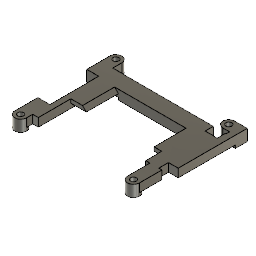
picooler (Autodesk Fusion 360 design; units mm, degrees)
Autodesk Fusion 360 part; units mm, degrees
sketch "Skizze1" plane through (0, 0, 0) normal (0, 0, 1) x (1, 0, 0)
  line L0 (0, 0) -> (65, 0)
  line L1 (65, 0) -> (65, 56)
  line L2 (65, 56) -> (0, 56)
  line L3 (0, 56) -> (0, 0)
  circle A0 centre (61.5, 52.5) radius 1.5
  circle A1 centre (3.5, 52.5) radius 1.5
  circle A2 centre (3.5, 3.5) radius 1.5
  circle A3 centre (61.5, 3.5) radius 1.5
  line L4 (3.5, 3.5) -> (61.5, 3.5) construction
  line L5 (61.5, 3.5) -> (61.5, 52.5) construction
  line L6 (61.5, 52.5) -> (3.5, 52.5) construction
  line L7 (3.5, 52.5) -> (3.5, 3.5) construction
  line L8 (9.5, 39.8) -> (56.2, 39.8) construction
  line L9 (56.2, 39.8) -> (56.2, 23.3) construction
  line L10 (56.2, 23.3) -> (9.5, 23.3) construction
  line L11 (9.5, 23.3) -> (9.5, 39.8) construction
  line L12 (18.5, 39.8) -> (18.5, 35.3) construction
  line L13 (18.5, 35.3) -> (9.5, 35.3) construction
  line L14 (19.5, 25) -> (33.5, 25) construction
  line L15 (33.5, 25) -> (33.5, 39) construction
  line L16 (33.5, 39) -> (19.5, 39) construction
  line L17 (19.5, 39) -> (19.5, 25) construction
  line L18 (7, 49.3) -> (17.5, 49.3) construction
  line L19 (17.5, 49.3) -> (17.5, 36.3) construction
  line L20 (17.5, 36.3) -> (7, 36.3) construction
  line L21 (7, 36.3) -> (7, 49.3) construction
  line L22 (52.2, 39.8) -> (52.2, 23.3) construction
  line L23 (17.5, 23.3) -> (17.5, 36.3) construction
  circle A4 centre (3.5, 52.5) radius 3.1
  circle A5 centre (61.5, 52.5) radius 3.1
  circle A6 centre (3.5, 3.5) radius 3.1
  circle A7 centre (61.5, 3.5) radius 3.1
  line L24 (6.6, 52.5) -> (0.4, 52.5) construction
  line L25 (0.4, 52.5) -> (0.4, 40.5)
  line L26 (0.4, 40.5) -> (6.6, 40.5)
  line L27 (6.6, 40.5) -> (6.6, 52.5)
  line L28 (61.5, 49.4) -> (68, 49.4)
  line L29 (68, 49.4) -> (68, 55.6)
  line L30 (68, 55.6) -> (61.5, 55.6)
  line L31 (61.5, 55.6) -> (61.5, 49.4) construction
  dimension "d1" = 65
  dimension "d2" = 56
  dimension "d3" = 49
  dimension "d4" = 3.5
  dimension "d5" = 4
  dimension "d6" = 3.5
  dimension "d7" = 3.5
  dimension "d8" = 3
  dimension "d9" = 3
  dimension "d10" = 3
  dimension "d11" = 3
  dimension "d12" = 46.7
  dimension "d13" = 16.5
  dimension "d14" = 4.5
  dimension "d15" = 9
  dimension "d16" = 14
  dimension "d17" = 14
  dimension "d18" = 17
  dimension "d19" = 19.5
  dimension "d20" = 10.5
  dimension "d21" = 13
  dimension "d22" = 6.7
  dimension "d23" = 7
  dimension "d24" = 2
  dimension "d25" = 1
  dimension "d26" = 1
  dimension "d27" = 1
  dimension "d28" = 4
  dimension "d29" = 8
  dimension "d30" = 6.2
  dimension "d31" = 6.2
  dimension "d32" = 6.2
  dimension "d33" = 6.2
  dimension "d36" = 12
  dimension "d37" = 6.5
  measures "d3" distance of L0.start
  measures "d4" distance of L0 L4
  measures "d5" distance of L2 L6
  measures "d6" distance of L1 L5
  measures "d7" distance of L3 L7
  measures "d8" diameter of A1
  measures "d9" diameter of A0
  measures "d10" diameter of A3
  measures "d11" diameter of A2
  measures "d12" distance of L0.start
  measures "d14" distance of L8 L13
  measures "d15" distance of L11 L12
  measures "d16" distance of L0.start
  measures "d17" distance of L14 L16
  measures "d18" distance of L2 L16
  measures "d19" distance of L3 L17
  measures "d22" distance of L2 L18
  measures "d23" distance of L3 L21
  measures "d24" distance of L17 L19
  measures "d25" distance of L12 L19
  measures "d26" distance of L12 L17
  measures "d27" distance of L13 L20
  measures "d28" distance of L9 L22
  measures "d29" distance of L11 L23
  measures "d30" diameter of A4
  measures "d31" diameter of A5
  measures "d32" diameter of A6
  measures "d33" diameter of A7
ref_plane "Arbeitsebene1" through (0, 0, 4) normal (0, 0, 1) x (1, 0, 0)
sketch "Skizze2" plane through (0, 0, 4) normal (0, 0, 1) x (1, 0, 0)
  line L0 (52.2, 39.8) -> (52.2, 23.3)
  line L1 (56.2, 39.8) -> (56.2, 23.3)
  line L2 (56.2, 23.3) -> (9.5, 23.3)
  line L3 (9.5, 39.8) -> (56.2, 39.8)
  line L4 (9.5, 23.3) -> (9.5, 39.8)
  line L5 (17.5, 23.3) -> (17.5, 36.3)
  line L6 (17.5, 49.3) -> (17.5, 36.3)
  line L7 (56.2, 39.8) -> (9.5, 39.8)
  line L8 (9.5, 39.8) -> (9.5, 47.8)
  line L9 (9.5, 47.8) -> (56.2, 47.8)
  line L10 (56.2, 47.8) -> (56.2, 39.8)
  line L11 (56.2, 47.8) -> (68, 47.8)
  line L12 (68, 47.8) -> (68, 15)
  line L13 (68, 15) -> (56.2, 15)
  line L14 (56.2, 15) -> (56.2, 47.8)
  line L15 (0, 0) -> (65, 0)
  line L16 (68, 49.4) -> (68, 55.6)
  line L17 (68, 15) -> (63, 15)
  line L18 (63, 15) -> (63, 20)
  line L19 (63, 20) -> (68, 20)
  line L20 (68, 20) -> (68, 15)
  line L21 (68, 49.4) -> (68, 47.8)
  line L22 (61.5, 49.4) -> (68, 49.4)
  line L23 (65, 0) -> (65, 56)
  line L24 (65, 47.8) -> (65, 49.4)
  line L25 (58.4, 47.8) -> (64.6, 47.8)
  line L26 (64.6, 47.8) -> (64.6, 43.5)
  line L27 (64.6, 43.5) -> (58.4, 43.5)
  line L28 (58.4, 43.5) -> (58.4, 47.8)
  circle A0 centre (61.5, 52.5) radius 3.1
  line L29 (58.4, 15) -> (64.6, 15)
  line L30 (64.6, 15) -> (64.6, 3.5)
  line L31 (64.6, 3.5) -> (58.4, 3.5)
  line L32 (58.4, 3.5) -> (58.4, 15)
  circle A1 centre (61.5, 3.5) radius 3.1
  line L33 (6.6, 40.5) -> (9.5, 40.5)
  line L34 (6.6, 40.5) -> (6.6, 52.5)
  line L35 (9.5, 47.8) -> (6.6, 47.8)
  line L36 (6.6, 3.5) -> (0.4, 3.5)
  line L37 (0.4, 3.5) -> (0.4, 15.5)
  line L38 (0.4, 15.5) -> (6.6, 15.5)
  line L39 (6.6, 15.5) -> (6.6, 3.5)
  circle A2 centre (3.5, 3.5) radius 3.1
  line L40 (3.5, 3.5) -> (61.5, 3.5)
  line L41 (6.6, 40.5) -> (6.6, 15.5)
  line L42 (9.5, 23.3) -> (9.5, 6.6)
  line L43 (6.6, 6.6) -> (9.5, 6.6)
  line L44 (6.6, 36.3) -> (9.5, 36.3)
  dimension "d45" = 8
  dimension "d50" = 15
  dimension "d52" = 20
  dimension "d53" = 5
  dimension "d70" = 9
  dimension "d81" = 12
  measures "d50" distance of L13 L15
  measures "d52" distance of L15 L19
  measures "d53" distance of L12 L18
extrude "Extrusion3" add sketch "Skizze2" along normal blind 2 contours L0 L1 L2 L3 L7 L14 | L2 L3 L4 L5 L6 L7 makes body 1 at (54.8667, 28.8, 4) makes body 2 at (12.1667, 28.8, 4)
chamfer "Fase1" distance 2 angle 45 1 edges at (17.5, 31.55, 6) measured on face at (12.1667, 28.8, 6) on bodies 2
extrude "Extrusion4" add sketch "Skizze2" along normal blind 2 contours L3 L6 L7 L9 L10 L14 | L3 L6 L7 L8 L9 bodies 1 2
extrude "Extrusion5" add sketch "Skizze2" against normal blind 3 contours L3 L6 L7 L9 L10 L14 bodies 1
extrude "Extrusion6" add sketch "Skizze2" along normal blind 2 and the other way blind 2.4 contours L1 L10 L11 L13 L14 L18 L19 L23 L26 L27 L28 L29 | L11 L12 L19 L23 bodies 1
extrude "Extrusion7" add sketch "Skizze1" along normal blind 6 separate body contours L1 A5 L28 L30 | L1 L28 L29 L30 | A5 makes body 3
extrude "Extrusion8" add sketch "Skizze1" along normal blind 6 separate body contours A4 | A4 L25 L26 L27 makes body 4
extrude "Extrusion9" add sketch "Skizze1" along normal blind 6 separate body contours A7 makes body 5
extrude "Extrusion10" add sketch "Skizze1" along normal blind 6 separate body contours A6 makes body 6
extrude "Extrusion11" add sketch "Skizze2" along normal blind 2 and the other way blind 2.4 contours L11 L21 L22 L23 L24 bodies 1 3
extrude "Extrusion12" add sketch "Skizze2" along normal blind 2 and the other way blind 2.4 contours L13 L17 L29 L30 L32 A1 bodies 1 5
extrude "Extrusion13" add sketch "Skizze2" against normal blind 1.7 contours L3 L6 L7 L8 L9 bodies 1
extrude "Extrusion14" add sketch "Skizze2" along normal blind 2 contours L8 L33 L34 L35 bodies 1 4
extrude "Extrusion15" add sketch "Skizze2" against normal blind 1.7 contours L8 L33 L34 L35 bodies 1
extrude "Extrusion16" add sketch "Skizze2" against normal blind 1.7 separate body contours L4 L8 L33 L41 L44 makes body 7
extrude "Extrusion17" add sketch "Skizze2" against normal blind 2.4 contours L4 L39 L41 L42 L43 L44 | L37 L38 L39 A2 bodies 6 1 7
extrude "Extrusion18" add sketch "Skizze2" along normal blind 2 contours L4 L8 L33 L41 L44 | L4 L39 L41 L42 L43 L44 | L37 L38 L39 A2 bodies 6
equation "d6 = d4"
equation "d7 = d4"
equation "d9 = d8"
equation "d10 = d8"
equation "d11 = d8"
